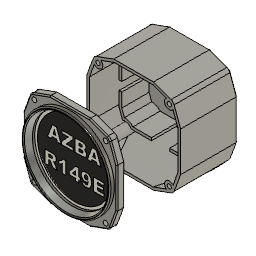
AZBA R149 Indicator (Autodesk Fusion 360 design; units mm, degrees)
Autodesk Fusion 360 part; units mm, degrees
note: some values were not read from the file. Chosen so that the rebuilt part matches the saved one: which bodies a step acts on; a direction; which face or edge a step refers to. Set by a fixed rule: which sketch regions a step uses.
sketch "Esquisse1" plane through (0, 0, 0) normal (0, 1, 0) x (1, 0, 0)
  line L0 (0, 0) -> (0, -82.5)
  line L1 (0, -82.5) -> (82.5, -82.5)
  line L2 (82.5, -82.5) -> (82.5, 0)
  line L3 (82.5, 0) -> (0, 0)
  line L4 (0, -82.5) -> (82.5, 0) construction
  line L5 (41.25, -41.25) -> (0, -41.25) construction
  circle A0 centre (9.9, -72.6) radius 2.1
  line L6 (5.6417, -74.1499) -> (0, -58.6493)
  line L7 (8.3501, -76.8583) -> (23.8507, -82.5)
  arc A1 (5.6417, -74.1499) -> (8.3501, -76.8583) centre (9.9, -72.6) ccw
  circle A2 centre (41.25, -41.25) radius 39
  circle A3 centre (41.25, -41.25) radius 35
  line L8 (9.9, -9.7939) -> (72.6, -9.7939) construction
  line L9 (72.6, -9.7939) -> (72.6, -72.6) construction
  line L10 (72.6, -72.6) -> (9.9, -72.6) construction
  line L11 (9.9, -72.6) -> (9.9, -9.7939) construction
  circle A4 centre (9.9, -72.6) radius 1.85
  line L12 (41.25, -41.25) -> (41.25, -9.7939) construction
  circle A5 centre (41.25, -19.7939) radius 4
  arc A6 (5.6417, -74.1499) -> (8.3501, -76.8583) centre (9.9, -72.6) ccw
  circle A7 centre (72.6, -72.6) radius 2.1
  circle A8 centre (72.6, -72.6) radius 1.85
  line L13 (76.8583, -74.1499) -> (82.5, -58.6493)
  arc A9 (74.1499, -76.8583) -> (76.8583, -74.1499) centre (72.6, -72.6) ccw
  line L14 (74.1499, -76.8583) -> (58.6493, -82.5)
  circle A10 centre (72.6, -9.9) radius 2.1
  circle A11 centre (72.6, -9.9) radius 1.85
  line L15 (74.1499, -5.6417) -> (58.6493, 0)
  arc A12 (76.8583, -8.3501) -> (74.1499, -5.6417) centre (72.6, -9.9) ccw
  line L16 (76.8583, -8.3501) -> (82.5, -23.8507)
  circle A13 centre (9.9, -9.9) radius 2.1
  circle A14 centre (9.9, -9.9) radius 1.85
  line L17 (5.6417, -8.3501) -> (0, -23.8507)
  arc A15 (8.3501, -5.6417) -> (5.6417, -8.3501) centre (9.9, -9.9) ccw
  line L18 (8.3501, -5.6417) -> (23.8507, 0)
  circle A16 centre (41.25, -41.25) radius 32.6
  point P0 (6.3645, -76.1355)
  dimension "d1" = 82.5
  dimension "d2" = 82.5
  dimension "d3" = 31.35
  dimension "d4" = 4.2
  dimension "d7" = 20
  dimension "d8" = 20
  dimension "d9" = 5
  dimension "d12" = 78
  dimension "d13" = 4
  dimension "d14" = 11
  dimension "d27" = 3.7
  dimension "d40" = 8
  dimension "d41" = 10
  dimension "d51" = 360
  dimension "d61" = 2.4
  text T0 "AZBA\nR149E" font "Arial Black" height 11 align centre middle in box 62.7 x 62.8061 at (9.9, -9.7939) x (1, 0) y (0, -1) spacing 1
  constraint coincident L0.start L3.end
  constraint parallel L0 L2
  constraint horizontal L1
  constraint midpoint L4 L5.start
  constraint midpoint L0 L5.end
  constraint coincident L4 A0.centre
  constraint coincident L4 P0
  constraint coincident L0 L6.end
  constraint coincident L1 L7.end
  constraint coincident P0 L6
  constraint coincident P0 L7
  constraint tangent L6 A1
  constraint tangent L7 A1
  constraint coincident L5.start A2.centre
  constraint concentric A2 A3
  constraint tangent A1 A6
  constraint concentric A0 A4
  constraint vertical L12
  constraint coincident L12 A5.centre
  constraint coincident L12.end
  constraint coincident A0.centre A1.centre
  constraint concentric A3 A16
  constraint coincident A0.centre
  constraint vertical L0
  constraint coincident L9.end
  measures "d1" distance of L1 L3
  measures "d2" distance of L0 L2
  measures "d3" horizontal distance of L5.start A0.centre
  measures "d4" diameter of A0
  measures "d7" angle of L1 L7
  measures "d8" angle of L0 L6
  measures "d9" distance of A0.centre P0
  measures "d12" diameter of A2
  measures "d13" distance of A2 A3
  measures "d27" diameter of A4
  measures "d40" diameter of A5
  measures "d41" distance of L12.end A5.centre
  measures "d61" distance of A3 A16
extrude "Extrusion1" add sketch "Esquisse1" along normal blind 2 contours L0 L1 L2 L3 L6 L7 A1 A6 L13 A9 L14 L15 A12 L16 L17 A15 L18 | A2 | A3 | A5 | A16 makes body 1
extrude "Extrusion6" add sketch "Esquisse1" against normal blind 4 contours L0 L1 L2 L3 L6 L7 A1 A6 L13 A9 L14 L15 A12 L16 L17 A15 L18 bodies 1
extrude "Extrusion7" add sketch "Esquisse1" against normal up to surface (8 mm away) separate body contours A2 makes body 2
chamfer "Chanfrein1" distance 6 distance2 2 1 edges at (8.6185, -8, 28.5935) measured on face at (76.2065, -5.3333, 42.9946) on bodies 2
extrude "Extrusion8" add sketch "Esquisse1" along normal up to surface (2 mm away) separate body text T0 makes body 3 at (26.5483, 0, 51.5967) makes body 4 at (42.8657, 0, 51.7292) makes body 5 at (54.0032, 0, 30.6717) makes body 6 at (32.5961, 0, 31.0348) makes body 7 at (43.9787, 0, 32.6956) makes body 8 at (16.4262, 0, 30.0169) makes body 9 at (61.5517, 0, 51.5967) makes body 10 at (36.5329, 0, 53.1374) makes body 11 at (59.0731, 0, 30.0819)
combine "Combiner4" operation cut target body 1 tool bodies 3 10 9 4 5 6 7 8 11 keep tools makes body 12 at (41.2225, 0.6667, 31.5951) makes body 13 at (19.6777, 2, 32.8957) makes body 14 at (41.4076, 2, 74.1773) makes body 15 at (51.8037, 2, 31.0495) makes body 16 at (46.3048, 2, 49.6383) makes body 17 at (46.1447, 2, 54.6081) makes body 18 at (59.3182, 0.6667, 52.0444)
extrude "Extrusion9" add sketch "Esquisse1" along normal up to surface (2 mm away) draft 30 separate body contours A3 makes body 19
combine "Combiner3" operation cut target body 14 tool bodies 19 keep tools makes body 20 at (19.5528, 2, 6.2187)
extrude "Extrusion6'" add sketch "Esquisse1" along normal blind 50 from surface at 2 separate body contours L0 L1 L2 L3 L6 L7 A1 A6 L13 A9 L14 L15 A12 L16 L17 A15 L18 | A0 | A2 | A3 | A5 | A7 | A10 | A13 | A16 makes body 21 in component "Component"
extrude "Extrusion7'" add sketch "Esquisse1" against normal blind 4.8 from surface at 52 contours A4 | A8 | A11 | A14 bodies 21 in component "Component"
sketch "Esquisse1 (2)" plane through (0, 0, 0) normal (-1, 0, 0) x (0, -1, 0) in component "Component"
  line L0 (-2, 23.8507) -> (-2, 58.6493)
  line L1 (-2, 58.6493) -> (-52, 58.6493)
  line L2 (-52, 58.6493) -> (-52, 23.8507)
  line L3 (-52, 23.8507) -> (-2, 23.8507)
  line L4 (-2, 0) -> (-2, 5.6417)
  line L5 (-2, 5.6417) -> (-52, 5.6417)
  line L6 (-52, 5.6417) -> (-52, 0)
  line L7 (-52, 0) -> (-2, 0)
  line L8 (-2, 0) -> (-65.2968, 11.1609)
  line L9 (-65.2968, 11.1609) -> (-65.2968, 0)
  line L10 (-65.2968, 0) -> (-2, 0)
  dimension "d74" = 10
  constraint coincident L4.start L7.end
  constraint perpendicular L7 L9
  constraint perpendicular L4 L10
  measures "d74" angle of L8 L10
extrude "Extrusion8'" cut sketch "Esquisse1 (2)" against normal through all contours L5 L6 L7 L8 L10 | L5 L6 L8 L9 L10 bodies 21 in component "Component"
shell "Coque3" thickness 2.4 removed faces 1 at (31.252, 2, 31.2194) on bodies 21 in component "Component"
extrude "Extrusion9'" cut sketch "Esquisse1" along normal through all contours A5 bodies 21 in component "Component"
fillet "Congé3" radius 1 1 faces at (30.8634, -8, 78.0495) on bodies 2
fillet "Congé4" radius 1 16 edges at (16.1004, -4, 79.6791) (6.6957, -4, 75.8043) (2.8209, -4, 66.3996) (41.25, -4, 82.5) (79.6791, -4, 66.3996) (75.8043, -4, 75.8043) (66.3996, -4, 79.6791) (82.5, -4, 41.25) (66.3996, -4, 2.8209) (75.8043, -4, 6.6957) (79.6791, -4, 16.1004) (41.25, -4, 0) (2.8209, -4, 16.1004) (6.6957, -4, 6.6957) (16.1004, -4, 2.8209) (0, -4, 41.25) on bodies 20
fillet "Congé2" radius 1 12 edges at (41.25, 52, 82.5) (66.3996, 52, 79.6791) (75.8043, 52, 75.8043) (79.6791, 52, 66.3996) (82.5, 52, 41.25) (79.764, 52, 16.3335) (41.25, 52, 8.8163) (2.736, 52, 16.3335) (0, 52, 41.25) (2.8209, 52, 66.3996) (6.6957, 52, 75.8043) (16.1004, 52, 79.6791) on bodies 21 in component "Component"
extrude "Extrusion10" add sketch "Esquisse1" against normal blind 8 from surface at 47.2 contours A4 | A8 | A11 | A14 bodies 21 in component "Component"
sketch "Esquisse3" plane through (0, 2, 0) normal (0, -1, 0) x (1, 0, 0) in component "Component"
  arc A0 (75.8605, 12.6261) -> (69.8739, 6.6395) centre (72.6, 9.9) ccw
  line L0 (69.8739, 6.6395) -> (58.3278, 2.437)
  line L1 (58.3278, 2.437) -> (24.1722, 2.437)
  line L2 (24.1722, 2.437) -> (12.6261, 6.6395)
  arc A1 (12.6261, 6.6395) -> (6.6395, 12.6261) centre (9.9, 9.9) ccw
  line L3 (6.6395, 12.6261) -> (2.4, 24.2739)
  line L4 (2.4, 24.2739) -> (2.4, 58.2261)
  line L5 (2.4, 58.2261) -> (6.6395, 69.8739)
  arc A2 (6.6395, 69.8739) -> (12.6261, 75.8605) centre (9.9, 72.6) ccw
  line L6 (12.6261, 75.8605) -> (24.2739, 80.1)
  line L7 (24.2739, 80.1) -> (58.2261, 80.1)
  line L8 (58.2261, 80.1) -> (69.8739, 75.8605)
  arc A3 (69.8739, 75.8605) -> (75.8605, 69.8739) centre (72.6, 72.6) ccw
  line L9 (75.8605, 69.8739) -> (80.1, 58.2261)
  line L10 (80.1, 58.2261) -> (80.1, 24.2739)
  line L11 (80.1, 24.2739) -> (75.8605, 12.6261)
  arc A4 (5.6417, 8.3501) -> (8.3501, 5.6417) centre (9.9, 9.9) ccw
  line L12 (8.3501, 5.6417) -> (23.8507, 0)
  line L13 (23.8507, 0) -> (58.6493, 0)
  line L14 (58.6493, 0) -> (74.1499, 5.6417)
  arc A5 (74.1499, 5.6417) -> (76.8583, 8.3501) centre (72.6, 9.9) ccw
  line L15 (76.8583, 8.3501) -> (82.5, 23.8507)
  line L16 (82.5, 23.8507) -> (82.5, 58.6493)
  line L17 (82.5, 58.6493) -> (76.8583, 74.1499)
  arc A6 (76.8583, 74.1499) -> (74.1499, 76.8583) centre (72.6, 72.6) ccw
  line L18 (74.1499, 76.8583) -> (58.6493, 82.5)
  line L19 (58.6493, 82.5) -> (23.8507, 82.5)
  line L20 (23.8507, 82.5) -> (8.3501, 76.8583)
  arc A7 (8.3501, 76.8583) -> (5.6417, 74.1499) centre (9.9, 72.6) ccw
  line L21 (5.6417, 74.1499) -> (0, 58.6493)
  line L22 (0, 58.6493) -> (0, 23.8507)
  line L23 (0, 23.8507) -> (5.6417, 8.3501)
  circle A8 centre (72.6, 72.6) radius 1.85
  circle A9 centre (9.9, 9.9) radius 1.85
  circle A10 centre (9.9, 72.6) radius 1.85
  circle A11 centre (72.6, 9.9) radius 1.85
  line L24 (41.25, 80.1) -> (41.25, 2.437) construction
  line L25 (28.05, 78.1) -> (28.05, 76.7)
  line L26 (28.05, 76.7) -> (30.45, 76.7)
  line L27 (30.45, 76.7) -> (30.45, 74.3)
  line L28 (30.45, 74.3) -> (25.65, 74.3)
  line L29 (25.65, 74.3) -> (25.65, 80.1)
  line L30 (28.05, 78.1) -> (30.45, 78.1)
  line L31 (30.45, 78.1) -> (30.45, 80.1)
  line L32 (30.45, 76.7) -> (30.45, 78.1) construction
  line L33 (52.05, 78.1) -> (52.05, 80.1)
  line L34 (54.45, 78.1) -> (52.05, 78.1)
  line L35 (54.45, 78.1) -> (54.45, 76.7)
  line L36 (54.45, 76.7) -> (52.05, 76.7)
  line L37 (52.05, 76.7) -> (52.05, 74.3)
  line L38 (52.05, 74.3) -> (56.85, 74.3)
  line L39 (56.85, 74.3) -> (56.85, 80.1)
  line L40 (2.4, 41.25) -> (80.1, 41.25) construction
  line L41 (4.8, 45.25) -> (7.2, 45.25)
  line L42 (4.8, 37.25) -> (7.2, 37.25)
  line L43 (75.3, 45.25) -> (77.7, 45.25)
  line L44 (75.3, 37.25) -> (77.7, 37.25)
  line L45 (20.5406, 76.1872) -> (21.3615, 73.9319)
  line L46 (61.9594, 76.1872) -> (61.1385, 73.9319)
  circle A12 centre (41.25, 19.7939) radius 4
  arc A13 (69.8739, 75.8605) -> (75.8605, 69.8739) centre (72.6, 72.6) ccw
  line L47 (69.8739, 75.8605) -> (58.2261, 80.1)
  line L48 (58.2261, 80.1) -> (24.2739, 80.1)
  line L49 (24.2739, 80.1) -> (12.6261, 75.8605)
  arc A14 (6.6395, 69.8739) -> (12.6261, 75.8605) centre (9.9, 72.6) ccw
  line L50 (6.6395, 69.8739) -> (2.4, 58.2261)
  line L51 (2.4, 58.2261) -> (2.4, 24.2739)
  line L52 (2.4, 24.2739) -> (6.6395, 12.6261)
  arc A15 (14.047, 10.8302) -> (6.6395, 12.6261) centre (9.9, 9.9) ccw
  line L53 (14.047, 10.8302) -> (68.453, 10.8302)
  arc A16 (75.8605, 12.6261) -> (68.453, 10.8302) centre (72.6, 9.9) ccw
  line L54 (75.8605, 12.6261) -> (80.1, 24.2739)
  line L55 (80.1, 24.2739) -> (80.1, 58.2261)
  line L56 (80.1, 58.2261) -> (75.8605, 69.8739)
  arc A17 (74.6203, 16.2357) -> (66.8439, 13.2302) centre (72.6, 9.9) ccw
  line L57 (15.6561, 13.2302) -> (66.8439, 13.2302)
  arc A18 (15.6561, 13.2302) -> (7.8797, 16.2357) centre (9.9, 9.9) ccw
  line L58 (4.8, 24.6971) -> (7.8797, 16.2357)
  line L59 (4.8, 57.8029) -> (4.8, 24.6971)
  line L60 (7.8797, 66.2643) -> (4.8, 57.8029)
  arc A19 (7.8797, 66.2643) -> (16.2357, 74.6203) centre (9.9, 72.6) ccw
  line L61 (24.6971, 77.7) -> (16.2357, 74.6203)
  line L62 (57.8029, 77.7) -> (24.6971, 77.7)
  line L63 (66.2643, 74.6203) -> (57.8029, 77.7)
  arc A20 (66.2643, 74.6203) -> (74.6203, 66.2643) centre (72.6, 72.6) ccw
  line L64 (77.7, 57.8029) -> (74.6203, 66.2643)
  line L65 (77.7, 24.6971) -> (77.7, 57.8029)
  line L66 (74.6203, 16.2357) -> (77.7, 24.6971)
  arc A21 (73.0501, 18.9388) -> (65.5952, 15.6302) centre (72.6, 9.9) ccw
  line L67 (16.9048, 15.6302) -> (65.5952, 15.6302)
  arc A22 (16.9048, 15.6302) -> (9.4499, 18.9388) centre (9.9, 9.9) ccw
  line L68 (7.2, 25.1202) -> (9.4499, 18.9388)
  line L69 (7.2, 57.3798) -> (7.2, 25.1202)
  line L70 (9.4499, 63.5612) -> (7.2, 57.3798)
  arc A23 (9.4499, 63.5612) -> (18.9388, 73.0501) centre (9.9, 72.6) ccw
  line L71 (25.1202, 75.3) -> (18.9388, 73.0501)
  line L72 (57.3798, 75.3) -> (25.1202, 75.3)
  line L73 (63.5612, 73.0501) -> (57.3798, 75.3)
  arc A24 (63.5612, 73.0501) -> (73.0501, 63.5612) centre (72.6, 72.6) ccw
  line L74 (75.3, 57.3798) -> (73.0501, 63.5612)
  line L75 (75.3, 25.1202) -> (75.3, 57.3798)
  line L76 (73.0501, 18.9388) -> (75.3, 25.1202)
  line L77 (33.25, 15.6302) -> (33.25, 13.2302)
  line L78 (49.25, 15.6302) -> (49.25, 13.2302)
  dimension "d90" = 2.4
  dimension "d91" = 2.4
  dimension "d92" = 2.4
  dimension "d93" = 13.2
  dimension "d94" = 2
  dimension "d95" = 1.4
  dimension "d111" = 4
  dimension "d112" = 4
  dimension "d113" = 4
  dimension "d114" = 4
  dimension "d121" = -2.4
  dimension "d122" = -2.4
  dimension "d123" = 4
  dimension "d124" = 4
  dimension "d125" = 8
  dimension "d126" = 8
  constraint midpoint L7 L24.start
  constraint perpendicular L7 L24
  constraint perpendicular L7 L25
  constraint perpendicular L25 L26
  constraint perpendicular L26 L27
  constraint perpendicular L27 L28
  constraint coincident L7 L29.end
  constraint vertical L29
  constraint perpendicular L25 L30
  constraint coincident L7 L31.end
  constraint perpendicular L7 L31
  constraint vertical L32
  constraint symmetric L24 L25.end L35.end
  constraint symmetric L24 L26.end L36.end
  constraint symmetric L24 L27.end L37.end
  constraint symmetric L24 L28.end L38.end
  constraint symmetric L24 L29.end L39.end
  constraint symmetric L24 L25.start L34.start
  constraint symmetric L24 L30.end L33.start
  constraint symmetric L24 L31.end L33.end
  constraint coincident L1 L24.end
  constraint midpoint L4 L40.start
  constraint midpoint L10 L40.end
  constraint coincident L41.end L69
  constraint coincident L41.start L59
  constraint coincident L42.start L59
  constraint coincident L42.end L69
  constraint coincident L44.start L75
  constraint coincident L43.start L75
  constraint coincident L43.end L65
  constraint coincident L44.end L65
  constraint coincident L45.end L71
  constraint perpendicular L45 L71
  constraint coincident L45.start L61
  constraint coincident L46.end L73
  constraint coincident L46.start L63
  constraint perpendicular L46 L73
  constraint coincident L67 L77.start
  constraint coincident L57 L77.end
  constraint perpendicular L57 L77
  constraint coincident L67 L78.start
  constraint coincident L57 L78.end
  constraint perpendicular L57 L78
  measures "d90" distance of L26.end L27.end
  measures "d91" distance of L25 L29
  measures "d92" distance of L25 L30.end
  measures "d93" horizontal distance of L24.start L25.start
  measures "d94" distance of L30.end L31.end
  measures "d95" distance of L25.end L25.start
  measures "d111" distance of L40 L41
  measures "d112" distance of L40 L42
  measures "d113" distance of L40 L44
  measures "d114" distance of L40 L43
  measures "d123" distance of L45.end L71.start
  measures "d124" distance of L46 L72.start
  measures "d125" distance of L24 L77
  measures "d126" distance of L24 L78
extrude "Extrusion11" add sketch "Esquisse3" along normal blind 16 from surface at -47.6 contours L7 L25 L29 L30 L31 L48 L62 | L25 L26 L27 L29 L62 L72 | L27 L28 L29 L72 bodies 21 in component "Component"
extrude "Extrusion12" add sketch "Esquisse3" along normal blind 26 from surface at -47.6 contours L7 L33 L34 L35 L39 L48 L62 | L35 L36 L37 L39 L62 L72 | L37 L38 L39 L72 bodies 21 in component "Component"
extrude "Extrusion14" add sketch "Esquisse3" along normal blind 24 from surface at -47.6 contours L43 L46 L63 A20 L64 L65 L73 A24 L74 L75 | L41 L45 L59 L60 A19 L61 L69 L70 A23 L71 | L44 A17 L57 L65 L66 A21 L67 L75 L76 L78 | L42 L57 A18 L58 L59 L67 A22 L68 L69 L77 bodies 21 in component "Component"
sketch "Esquisse4" plane through (0, 52, 0) normal (0, 1, 0) x (-1, 0, 0)
  circle A0 centre (-41.25, 19.7939) radius 4
  line L0 (-1, 58.473) -> (-6.5814, 73.8079)
  arc A1 (-6.5814, 73.8079) -> (-8.6921, 75.9186) centre (-9.9, 72.6) ccw
  line L1 (-8.6921, 75.9186) -> (-24.027, 81.5)
  line L2 (-24.027, 81.5) -> (-58.473, 81.5)
  line L3 (-58.473, 81.5) -> (-73.8079, 75.9186)
  arc A2 (-73.8079, 75.9186) -> (-75.9186, 73.8079) centre (-72.6, 72.6) ccw
  line L4 (-75.9186, 73.8079) -> (-81.5, 58.473)
  line L5 (-81.5, 58.473) -> (-81.5, 24.027)
  line L6 (-81.5, 24.027) -> (-76.2692, 9.6554)
  line L7 (-76.2692, 9.6554) -> (-6.2308, 9.6554)
  line L8 (-6.2308, 9.6554) -> (-1, 24.027)
  line L9 (-1, 24.027) -> (-1, 58.473)
  circle A3 centre (-19.25, 19.7939) radius 1
  circle A4 centre (-19.25, 19.7939) radius 2
  circle A5 centre (-19.25, 19.7939) radius 3
  line L10 (-19.25, 19.7939) -> (-21.3713, 21.9152)
  line L11 (-19.25, 19.7939) -> (-21.3713, 17.6726)
  line L12 (-13.25, 19.2939) -> (-25.25, 19.2939)
  line L13 (-25.25, 19.2939) -> (-25.25, 20.2939)
  line L14 (-25.25, 20.2939) -> (-13.25, 20.2939)
  line L15 (-13.25, 20.2939) -> (-13.25, 19.2939)
  line L16 (-13.25, 19.2939) -> (-25.25, 20.2939) construction
  line L17 (-25.25, 19.2939) -> (-13.25, 20.2939) construction
  line L18 (-11.25, 20.2939) -> (-7.25, 20.2939)
  line L19 (-7.25, 20.2939) -> (-7.25, 19.2939)
  line L20 (-7.25, 19.2939) -> (-11.25, 19.2939)
  line L21 (-11.25, 19.2939) -> (-11.25, 20.2939)
  line L22 (-13.25, 20.2939) -> (-11.25, 20.2939) construction
  line L23 (-31.25, 20.2939) -> (-27.25, 20.2939)
  line L24 (-27.25, 20.2939) -> (-27.25, 19.2939)
  line L25 (-27.25, 19.2939) -> (-31.25, 19.2939)
  line L26 (-31.25, 19.2939) -> (-31.25, 20.2939)
  line L27 (-27.25, 20.2939) -> (-25.25, 20.2939) construction
  line L28 (-27.25, 19.2939) -> (-25.25, 19.2939) construction
  line L29 (-29.75, 21.7939) -> (-28.75, 21.7939)
  line L30 (-28.75, 21.7939) -> (-28.75, 17.7939)
  line L31 (-28.75, 17.7939) -> (-29.75, 17.7939)
  line L32 (-29.75, 17.7939) -> (-29.75, 21.7939)
  line L33 (-31.25, 20.2939) -> (-27.25, 19.2939) construction
  line L34 (-29.75, 17.7939) -> (-28.75, 21.7939) construction
  line L35 (-31.25, 19.7939) -> (-41.25, 19.7939) construction
  line L36 (-31.2218, 24.7939) -> (-7.2782, 24.7939) construction
  line L37 (-7.2782, 24.7939) -> (-7.2782, 31.459) construction
  line L38 (-7.2782, 31.459) -> (-31.2218, 31.459) construction
  line L39 (-31.2218, 31.459) -> (-31.2218, 24.7939) construction
  line L40 (-19.25, 24.7939) -> (-19.25, 19.7939) construction
  point P0 (-19.25, 19.7939)
  point P1 (-29.25, 19.7939)
  dimension "d130" = 2
  dimension "d132" = 4
  dimension "d133" = 1
  dimension "d136" = 12
  dimension "d137" = 1
  dimension "d138" = 45
  dimension "d139" = 45
  dimension "d140" = 4
  dimension "d141" = 1
  dimension "d142" = 2
  dimension "d143" = 1
  dimension "d144" = 4
  dimension "d145" = 4
  dimension "d146" = 2
  dimension "d147" = 10
  dimension "d148" = 4
  dimension "d149" = 0
  dimension "d150" = 5
  text T0 "5 Volts" font "Arial Black" height 4 align centre middle in box 23.9436 x 6.665 at (-31.2218, 24.7939) x (1, 0) y (0, 1) spacing 1
  constraint concentric A3 A4
  constraint concentric A3 A5
  constraint coincident P0 A3.centre
  constraint coincident A5 L10.end
  constraint coincident A5 L11.end
  constraint horizontal L12
  constraint perpendicular L12 L13
  constraint parallel L12 L14
  constraint parallel L13 L15
  constraint coincident L16 P0
  constraint coincident L17 P0
  constraint horizontal L18
  constraint vertical L19
  constraint horizontal L20
  constraint vertical L21
  constraint horizontal L22
  constraint horizontal L23
  constraint vertical L24
  constraint horizontal L25
  constraint vertical L26
  constraint horizontal L27
  constraint horizontal L28
  constraint horizontal L29
  constraint vertical L30
  constraint horizontal L31
  constraint vertical L32
  constraint midpoint L34 P1
  constraint midpoint L33 P1
  constraint midpoint L26 L35.start
  constraint coincident A0.centre L35.end
  constraint horizontal L35
  constraint midpoint L36 L40.start
  constraint vertical L40
  constraint horizontal L38
  measures "d130" diameter of A3
  measures "d132" diameter of A4
  measures "d133" distance of A4 A5
  measures "d136" distance of L13.end L14.end
  measures "d137" distance of L12.end L13.end
  measures "d138" angle of L10 L14
  measures "d139" angle of L11 L12
  measures "d140" distance of L18.start L18.end
  measures "d141" distance of L18.start L20.end
  measures "d142" distance of L14.end L18.start
  measures "d143" distance of L29.start L29.end
  measures "d144" distance of L29.start L31.end
  measures "d145" distance of L23.start L23.end
  measures "d146" distance of L12.end L24.end
  measures "d147" distance of L35.start A0.centre
  measures "d150" distance of L40.start P0
extrude "Extrusion15" cut sketch "Esquisse4" sketch "Esquisse4" against normal blind 0.4 contours A3 L10 L11 L12 L14 | A3 L10 L14 | A3 L11 L12 | A3 L10 L14 | A3 L10 L11 L12 L14 | A4 A5 L12 L14 | A4 A5 L10 L14 | A3 L11 L12 | A4 A5 L11 L12 | A3 A4 L12 L14 | A5 L12 L14 L15 | A4 A5 L12 L14 | A5 L12 L13 L14 | L18 L19 L20 L21 | L23 L25 L26 L32 | L23 L29 L30 L32 | L23 L25 L30 L32 | L23 L24 L25 L30 | L25 L30 L31 L32 picked at (-16.9571, 21.145) picked at (-16.9571, 18.4429) picked at (-20.9104, 19.685) of sketch 2 text T0 bodies 21 in component "Component"
move_body "Déplacer3" bodies 21 to x (1, 0, 0) y (0, 1, 0) z (0, 0, 1) at (0, 50, 0) in component "Component"
component "Component" placed x (1, 0, 0) y (0, 1, 0) z (0, 0, 1) at (0, 0, 0)
equation "d2 = d1"
equation "d3 = ( 62.7 / 2 ) * 1 mm"
equation "d8 = d7"
equation "d15 = Text1-Text"
equation "d90 = d91"
equation "d92 = d91"
equation "d93 = ( ( 26 / 2 ) * 1 mm ) + 0.2 * 1 mm"
equation "d112 = d111"
equation "d113 = d111"
equation "d114 = d111"
equation "d123 = d111"
equation "d124 = d111"
equation "d125 = d111 * 2"
equation "d126 = d111 * 2"
equation "d139 = d138"
equation "d146 = d142"
equation "d149 = '5 Volts'"
